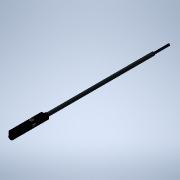
# Autodesk Inventor part: 551373 SMT-10M-PS-24V-E-2.5-L-OE
Saved by Autodesk Inventor 2021 (Build 250183000, 183)
## iProperties
Created: 2025-06-05
Part Number: 551373 SMT-10M-PS-24V-E-2.5-L-OE
Material: Generic
Catalog Web Link: www.cadenas.de
Description: SMT-10M (Schalter)-Proximity sensor
Vendor: FESTO
Document SubType Name: Modeling
Designer: psAdmin
Manufacturer: FESTO
Mass: 0.529111 g
Surface Area: 8.90335 cm^2
Volume: 0.529111 cm^3
Density: 1 g/cm^3
Appearance: PSOLRGB-191-191-191
Category: PARTsolutions
Company: FESTO
Title: 551373 SMT-10M-PS-24V-E-2.5-L-OE
Author: Cadenas PARTsolutions
Comments: Proximity sensor
PSOL_IDENT_0: {$CADENAS_DATA/23d-libs/festo/parts/s/smt/parts/smt_10m.prj},233 {VTYP=3D},{NB=551373 SMT-10M-PS-24V
PSOL_IDENT_1: -E-2.5-L-OE},{LINA=551373 SMT-10M-PS-24V-E-2.5-L-OE},{NN=SMT-10M (Schalter)},{DATE=30.08.2021 11:52:
PSOL_IDENT_2: 31},{GEOMDATE=03.04.2020 09:11:53},{VERSION=},{LINEID=10},{WBVAR=TNR,SA,LL,KA,AT},{WBNUMERIC=LL}  {N
PSOL_IDENT_3: B=551373 SMT-10M-PS-24V-E-2.5-L-OE},{LINA=551373 SMT-10M-PS-24V-E-2.5-L-OE},{KT=DUMMY},{TNR=551373},
PSOL_IDENT_4: {TYP=SMT-10M},{L=20.950},{L2=5.600},{L3=9.050},{L4=10.900},{SA=PS},{LL=2.5},{LL1=[0.2:5/0.1], [5:30/
PSOL_IDENT_5: 0.5]},{KA=L},{AT=OE},{L1=80}
NB: 551373 SMT-10M-PS-24V-E-2.5-L-OE
NN: SMT-10M (Schalter)
NT: Proximity sensor
NBSYN: $TNR. $TYP.-$SA.-24V-E-$LL.-$KA.-$AT.
LINA: 551373 SMT-10M-PS-24V-E-2.5-L-OE
CATALOG: Festo
TNR: 551373
TYP: SMT-10M
L: 20.95
L2: 5.6
L3: 9.05
L4: 10.9
SA: PS
LL: 2.5
LL1: [0.2:5/0.1], [5:30/0.5]
KA: L
AT: OE
SUPPLIER: FESTO
ARTICLENO: 551373 SMT-10M-PS-24V-E-2.5-L-OE
BOMINFO: 551373 SMT-10M-PS-24V-E-2.5-L-OE
CREATOR: CADENAS GmbH
Autodesk Inventor part; units mm, degrees
sketch "Sketch_1" plane through (0, 0, 0) normal (0, 0, 1) x (1, 0, 0)
  arc A0 (-1.475, 0.8083) -> (1.475, 0.8083) centre (0, 1.75) ccw
  line L0 (1.475, 0.8083) -> (1.4438, 4.387)
  arc A1 (1.4438, 4.387) -> (-1.4438, 4.387) centre (0, -0.4) ccw
  line L1 (-1.4438, 4.387) -> (-1.475, 0.8083)
  constraints: 4 end point, 4 point on circle, 2 centre point
extrude "Extrusion1" add sketch "Sketch_1" along normal blind 20.95
sketch "Sketch_2" plane through (0, 0, 0) normal (1, 0, 0) x (0, 1, 0)
  line L0 (2.3501, 9.8094) -> (1.5, 9.5)
  line L1 (1.5, 9.5) -> (1.5, 5.9)
  line L2 (1.5, 5.9) -> (2.3501, 5.5906)
  line L3 (2.3501, 5.5906) -> (3.2, 5.65)
  line L4 (3.2, 5.65) -> (3.2, 9.75)
  line L5 (3.2, 9.75) -> (2.3501, 9.8094)
  constraints: 12 end point
extrude "Extrusion2" cut sketch "Sketch_2" along normal mid plane 6
sketch "Sketch_3" plane through (0, 1.4, 0) normal (0, 1, 0) x (1, 0, 0)
  line L0 (-3, -11) -> (3, -11)
  line L1 (3, -11) -> (3, -5)
  line L2 (3, -5) -> (-3, -5)
  line L3 (-3, -5) -> (-3, -11)
  line L4 (-2, -6.6) -> (-2, -9.75)
  line L5 (-2, -9.75) -> (0.525, -9.75)
  line L6 (0.525, -9.75) -> (0.6286, -9.0961)
  line L7 (0.6286, -9.0961) -> (1.0258, -8.8)
  line L8 (1.0258, -8.8) -> (2, -8.8)
  line L9 (2, -8.8) -> (2, -5.65)
  line L10 (2, -5.65) -> (-0.525, -5.65)
  line L11 (-0.525, -5.65) -> (-0.6286, -6.3039)
  line L12 (-0.6286, -6.3039) -> (-1.0258, -6.6)
  line L13 (-1.0258, -6.6) -> (-2, -6.6)
  constraints: 28 end point
extrude "Extrusion3" add sketch "Sketch_3" along normal blind 2.8
sketch "Sketch_4" plane through (0, 0, 0) normal (0, 0, 1) x (1, 0, 0)
  line L0 (-3, -1) -> (3, -1)
  line L1 (3, -1) -> (3, 7)
  line L2 (3, 7) -> (-3, 7)
  line L3 (-3, 7) -> (-3, -1)
  line L4 (-1.4821, 0) -> (1.4821, 0)
  line L5 (1.4821, 0) -> (1.4253, 6.5)
  line L6 (1.4253, 6.5) -> (-1.4253, 6.5)
  line L7 (-1.4253, 6.5) -> (-1.4821, 0)
  constraints: 16 end point
extrude "Extrusion4" cut sketch "Sketch_4" along normal blind 20.95
sketch "Sketch_5" plane through (0, 1.5, 0) normal (0, 1, 0) x (1, 0, 0)
  line L0 (-1.45, -7.7) -> (-1.45, -8.18)
  arc A0 (-1.45, -8.18) -> (-0.8232, -9.45) centre (0.15, -8.18) ccw
  line L1 (-0.8232, -9.45) -> (0.2938, -9.45)
  arc A1 (0.2938, -9.45) -> (0.5901, -9.1969) centre (0.2938, -9.15) ccw
  line L2 (0.5901, -9.1969) -> (0.5962, -9.1584)
  arc A2 (0.7395, -8.9473) -> (0.5962, -9.1584) centre (0.8925, -9.2053) ccw
  arc A3 (0.7395, -8.9473) -> (1.45, -7.7) centre (0, -7.7) ccw
  line L3 (1.45, -7.7) -> (1.45, -7.22)
  arc A4 (1.45, -7.22) -> (0.8232, -5.95) centre (-0.15, -7.22) ccw
  line L4 (0.8232, -5.95) -> (-0.2938, -5.95)
  arc A5 (-0.2938, -5.95) -> (-0.5901, -6.2031) centre (-0.2938, -6.25) ccw
  line L5 (-0.5901, -6.2031) -> (-0.5962, -6.2416)
  arc A6 (-0.7395, -6.4527) -> (-0.5962, -6.2416) centre (-0.8925, -6.1947) ccw
  arc A7 (-0.7395, -6.4527) -> (-1.45, -7.7) centre (0, -7.7) ccw
  constraints: 16 point on circle, 12 end point, 8 centre point
extrude "Extrusion5" add sketch "Sketch_5" along normal blind 0.3
sketch "Sketch_6" plane through (0, 1.8, 0) normal (0, 1, 0) x (1, 0, 0)
  arc A0 (-1.8279, -8.2184) -> (-0.3332, -9.5706) centre (0, -7.7) ccw
  line L0 (-0.3332, -9.5706) -> (-0.0383, -9.1495)
  arc A1 (-0.0383, -9.1495) -> (1.4498, -7.7216) centre (0, -7.7) ccw
  line L1 (1.4498, -7.7216) -> (1.8279, -7.1816)
  arc A2 (1.8279, -7.1816) -> (0.3332, -5.8294) centre (0, -7.7) ccw
  line L2 (0.3332, -5.8294) -> (0.0383, -6.2505)
  arc A3 (0.0383, -6.2505) -> (-1.4498, -7.6784) centre (0, -7.7) ccw
  line L3 (-1.4498, -7.6784) -> (-1.8279, -8.2184)
  constraints: 8 end point, 8 point on circle, 4 centre point
extrude "Extrusion6" add sketch "Sketch_6" along normal blind 0.8
sketch "Sketch_7" plane through (0, 0, 7.7) normal (0, 0, 1) x (1, 0, 0)
  line L0 (0, 1.8) -> (0, 2.6)
  line L1 (1.8295, 1.8) -> (1.9176, 1.8)
  line L2 (1.9176, 1.8) -> (1.9176, 2.3)
  line L3 (1.9176, 2.3) -> (1.8295, 1.8)
  constraints: 8 end point
revolve "Revolution1" cut sketch "Sketch_7" angle 83 about axis through (0, 1.8, 7.7) along (0, 1, 0)
sketch "Sketch_8" plane through (0, 0, 7.7) normal (0, 0, 1) x (1, 0, 0)
  line L0 (0, 2.6) -> (0, 1.8)
  line L1 (-1.9176, 2.3) -> (-1.9176, 1.8)
  line L2 (-1.9176, 1.8) -> (-1.8295, 1.8)
  line L3 (-1.8295, 1.8) -> (-1.9176, 2.3)
  constraints: 8 end point
revolve "Revolution2" cut sketch "Sketch_8" angle 83 about axis through (0, 2.6, 7.7) along (0, 1, 0)
sketch "Sketch_9" plane through (0, 0, 7.7) normal (0, 0, 1) x (1, 0, 0)
  line L0 (0, 1.8) -> (0, 4.7)
  line L1 (0, 4.7) -> (1.1, 4.7)
  line L2 (1.1, 4.7) -> (1.2, 4.6)
  line L3 (1.2, 4.6) -> (1.2, 3.25)
  line L4 (1.2, 3.25) -> (1.1423, 3.15)
  line L5 (1.1423, 3.15) -> (0.715, 3.15)
  line L6 (0.715, 3.15) -> (0.715, 2.95)
  line L7 (0.715, 2.95) -> (0.7775, 2.95)
  line L8 (0.7775, 2.95) -> (0.9, 2.8275)
  line L9 (0.9, 2.8275) -> (0.9, 1.9225)
  line L10 (0.9, 1.9225) -> (0.7775, 1.8)
  line L11 (0.7775, 1.8) -> (0, 1.8)
  line L12 (0, 1.8) -> (0, 4.7)
  constraints: 26 end point
revolve "Revolution3" add sketch "Sketch_9" angle 360 about axis through (0, 1.8, 7.7) along (0, -1, 0)
thread "Thread1" size "M1.8x0.2" class "6g" standard "ISO Metric profile" length 0.905
sketch "Sketch_10" plane through (0, 4.7, 0) normal (0, 1, 0) x (1, 0, 0)
  line L0 (-0.75, -8.133) -> (0, -8.566)
  line L1 (0, -8.566) -> (0.75, -8.133)
  line L2 (0.75, -8.133) -> (0.75, -7.267)
  line L3 (0.75, -7.267) -> (0, -6.834)
  line L4 (0, -6.834) -> (-0.75, -7.267)
  line L5 (-0.75, -7.267) -> (-0.75, -8.133)
  constraints: 12 end point
extrude "Extrusion7" cut sketch "Sketch_10" against normal blind 1
sketch "Sketch_11" plane through (0, 3, 0) normal (0, 1, 0) x (1, 0, 0)
  line L0 (-1.35, -16.9) -> (1.35, -16.9)
  line L1 (1.35, -16.9) -> (1.35, -16.6)
  line L2 (1.35, -16.6) -> (0.15, -16.6)
  line L3 (0.15, -16.6) -> (0.15, -16)
  line L4 (0.15, -16) -> (-0.15, -16)
  line L5 (-0.15, -16) -> (-0.15, -16.6)
  line L6 (-0.15, -16.6) -> (-1.35, -16.6)
  line L7 (-1.35, -16.6) -> (-1.35, -16.9)
  constraints: 16 end point
extrude "Extrusion8" add sketch "Sketch_11" along normal blind 3
sketch "Sketch_12" plane through (0, 0, 16.75) normal (0, 0, 1) x (1, 0, 0)
  line L0 (-2, 7) -> (-2, 4.4)
  arc A0 (2, 4.4) -> (-2, 4.4) centre (0, -0.4) ccw
  line L1 (2, 4.4) -> (2, 7)
  line L2 (2, 7) -> (-2, 7)
  constraints: 6 end point, 2 point on circle, 1 centre point
extrude "Extrusion9" cut sketch "Sketch_12" along normal mid plane 6
sketch "Sketch_13" plane through (0, 0, 0) normal (0, 0, 1) x (1, 0, 0)
  arc A0 (-1.475, 0.8083) -> (1.475, 0.8083) centre (0, 1.75) ccw
  line L0 (1.475, 0.8083) -> (1.4607, 2.4506)
  arc A1 (1.4607, 2.4506) -> (-1.4607, 2.4506) centre (0, 2.338) ccw
  line L1 (-1.4607, 2.4506) -> (-1.475, 0.8083)
  constraints: 4 end point, 4 point on circle, 2 centre point
extrude "Extrusion10" add sketch "Sketch_13" against normal blind 2
sketch "Sketch_15" plane through (0, 0, 18.6) normal (0, 0, 1) x (1, 0, 0)
  line L0 (-1.05, 5.46) -> (-1.05, 4.46)
  line L1 (-1.05, 4.46) -> (-0.375, 4.46)
  line L2 (-0.375, 4.46) -> (-0.375, 5.46)
  line L3 (-0.375, 5.46) -> (-1.05, 5.46)
  constraints: 8 end point
extrude "Extrusion11" cut sketch "Sketch_15" along normal mid plane 1.4
sketch "Sketch_16" plane through (0, 0, 0) normal (1, 0, 0) x (0, 1, 0)
  line L0 (2.3, -80) -> (2.3, 0)
  line L1 (2.3, 0) -> (3.375, 0)
  line L2 (3.375, 0) -> (3.375, -80)
  line L3 (3.375, -80) -> (2.3, -80)
  line L4 (2.3, -80) -> (2.3, 0)
  constraints: 10 end point
revolve "Revolution4" add sketch "Sketch_16" angle 360 about axis through (0, 2.3, -80) along (0, 0, -1)
sketch "Sketch_19" plane through (0, 0, -80) normal (0, 0, 1) x (1, 0, 0)
  line L0 (-2, 1) -> (2, 1)
  line L1 (2, 1) -> (2, 5)
  line L2 (2, 5) -> (-2, 5)
  line L3 (-2, 5) -> (-2, 1)
  circle A0 centre (0.3464, 2.1) radius 0.3
  circle A1 centre (0, 2.7) radius 0.3
  circle A2 centre (-0.3464, 2.1) radius 0.3
  constraints: 8 end point, 3 centre point
extrude "Extrusion12" cut sketch "Sketch_19" along normal blind 10
ref_plane "ANBAU_XY" through (0, 0, 0) normal (0, 0, -1) x (1, 0, 0)
ref_plane "ANBAU_YZ" through (0, 0, 0) normal (1, 0, 0) x (0, -1, 0)
ref_plane "ANBAU_ZX" through (0, 0, 0) normal (0, -1, 0) x (0, 0, -1)
ref_plane "ASCF1_XY" through (0, 2.3, -10) normal (0, 0, -1) x (1, 0, 0)
ref_plane "ASCF1_YZ" through (0, 2.3, -10) normal (1, 0, 0) x (0, -1, 0)
ref_plane "ASCF1_ZX" through (0, 2.3, -10) normal (0, -1, 0) x (0, 0, -1)
ref_plane "ASCF2_XY" through (0, 2.3, -60) normal (0, 0, 1) x (1, 0, 0)
ref_plane "ASCF2_YZ" through (0, 2.3, -60) normal (1, 0, 0) x (0, 1, 0)
ref_plane "ASCF2_ZX" through (0, 2.3, -60) normal (0, 1, 0) x (0, 0, 1)
ref_plane "CLIP_XY" through (0, 2.3, -32.5) normal (0, 0, 1) x (1, 0, 0)
ref_plane "CLIP_YZ" through (0, 2.3, -32.5) normal (1, 0, 0) x (0, 1, 0)
ref_plane "CLIP_ZX" through (0, 2.3, -32.5) normal (0, 1, 0) x (0, 0, 1)
ref_plane "FDT_NUT_XY" through (0, 0, 20.95) normal (0, -1, 0) x (1, 0, 0)
ref_plane "FDT_NUT_YZ" through (0, 0, 20.95) normal (1, 0, 0) x (0, 0, 1)
ref_plane "FDT_NUT_ZX" through (0, 0, 20.95) normal (0, 0, 1) x (0, -1, 0)
body "Solid1"
